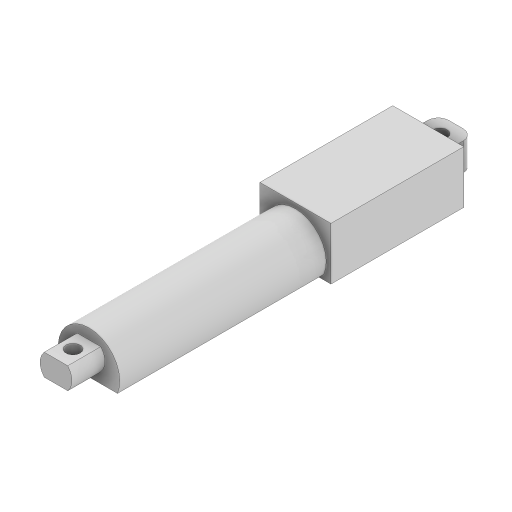
# Autodesk Inventor part: actuator
Saved by Autodesk Inventor 2023 (Build 270158000, 158)
## iProperties
Created: 2023-05-17
Part Number: actuator
Material: Generic
Document SubType Name: Modeling
Designer: Juyoung Han
Density: 1 g/cm^3
Appearance: Default
Author: Juyoung Han
Autodesk Inventor part; units mm, degrees
ref_plane "YZ Plane" through (0, 0, 0) normal (1, 0, 0) x (0, 1, 0)
ref_plane "XZ Plane" through (0, 0, 0) normal (0, 1, 0) x (-1, 0, 0)
ref_plane "XY Plane" through (0, 0, 0) normal (0, 0, 1) x (1, 0, 0)
sketch "Sketch1" plane through (0, 0, 0) normal (0, 0, 1) x (1, 0, 0)
  line L0 (0, 0) -> (20, 0)
  line L1 (20, 0) -> (20, -14.8)
  line L2 (20, -14.8) -> (0, -14.8)
  line L3 (0, -14.8) -> (0, 0)
  dimension "d0" = 20
  dimension "d1" = 14.8
  constraints: 8 end point, 2 parallel, 1 horizontal, 1 perpendicular
  measures "d0" distance of L1.end L2.end
  measures "d1" distance of L0.end L1.end
extrude "Extrusion1" add sketch "Sketch1" along normal blind 37.4
sketch "Sketch2" plane through (0, 0, 37.4) normal (0, 0, 1) x (1, 0, 0)
  line L0 (0, 0) -> (0, -14.8) projected
  line L1 (20, 0) -> (0, 0) projected
  line L2 (2, -13.4) -> (18, -13.4)
  arc A0 (18, -13.4) -> (2, -13.4) centre (10, -10.0667) ccw
  point P0 (10, -7.4)
  point P1 (10, -13.4)
  constraints: 2 end point, 2 point on circle, 1 centre point, 1 horizontal, 1 midpoint
extrude "Extrusion2" add sketch "Sketch2" along normal blind 58.1
sketch "Sketch3" plane through (0, 0, 95.5) normal (0, 0, 1) x (1, 0, 0)
  arc A0 (18, -13.4) -> (2, -13.4) centre (10, -10.0667) ccw projected
  line L0 (2, -13.4) -> (18, -13.4) projected
  line L1 (2, -13.4) -> (2, -13.4)
  line L2 (2, -13.4) -> (2, -13.4) construction
  line L3 (10, -13.4) -> (22, -13.4) construction
  line L4 (18, -13.4) -> (2, -13.4) projected
  line L5 (0, -14.8) -> (20, -14.8) projected
  line L6 (6.6913, -4.35) -> (13.3087, -4.35)
  line L7 (6.6913, -10.45) -> (13.3087, -10.45)
  arc A1 (6.6913, -4.35) -> (6.6913, -10.45) centre (10, -7.4) ccw
  arc A2 (13.3087, -10.45) -> (13.3087, -4.35) centre (10, -7.4) ccw
  point P0 (0, 0)
  dimension "d12" = 90
  constraints: 10 end point, 5 point on circle, 2 centre point, 2 horizontal, 1 midpoint, 1 perpendicular, 1 point on line
  measures "d12" angle of L2 L1
extrude "Extrusion3" add sketch "Sketch3" along normal blind 9.3 contours L6 A2 L7 A1
sketch "Sketch4" plane through (6.6913, -4.35, 95.5) normal (0, 1, 0) x (1, 0, 0)
  circle A0 centre (3.3087, -4.5) radius 2
  line L0 (-5.358, 0) -> (11.9754, 0) projected
  point P0 (-6.6913, 95.5)
  point P1 (11.3087, 0)
  point P2 (-4.6913, 0)
  dimension "d21" = 4
  dimension "d22" = 4.5
  constraints: 1 centre point
  measures "d21" diameter of A0
  measures "d22" distance from line of L0 A0.centre
extrude "Extrusion4" cut sketch "Sketch4" against normal through all
sketch "Sketch5" plane through (0, 0, 0) normal (0, 0, -1) x (-1, 0, 0)
  line L0 (-15, -3.5) -> (-5, -3.5)
  line L1 (-5, -3.5) -> (-5, -11.3)
  line L2 (-5, -11.3) -> (-15, -11.3)
  line L3 (-15, -11.3) -> (-15, -3.5)
  line L4 (-15, -3.5) -> (-5, -11.3) construction
  line L5 (-5, -3.5) -> (-15, -11.3) construction
  line L6 (-20, 0) -> (0, 0) projected
  line L7 (0, -14.8) -> (-20, -14.8) projected
  line L8 (0, 0) -> (0, -14.8) projected
  line L9 (-20, 0) -> (0, 0) projected
  line L10 (-20, -14.8) -> (-20, 0) projected
  point P0 (-10, -7.4)
  point P1 (0, -7.4)
  point P2 (-10, -7.4)
  dimension "d25" = 7.8
  dimension "d26" = 10
  dimension "d27" = 10
  constraints: 12 end point, 4 midpoint, 2 parallel, 1 horizontal, 1 perpendicular
  measures "d25" distance of L0.end L1.end
  measures "d26" distance of point (0, -7.4) point (-10, -7.4)
  measures "d27" distance of L1.end L2.end
extrude "Extrusion5" add sketch "Sketch5" along normal blind 7.8 contours L0 L1 L2 L3
sketch "Sketch6" plane through (5, -3.5, 0) normal (0, 1, 0) x (1, 0, 0)
  circle A0 centre (5, 3.3) radius 2
  line L0 (0, 7.8) -> (10, 7.8) projected
  line L1 (0, 0) -> (0, 7.8) projected
  point P0 (-5, 0)
  point P1 (5, 7.8)
  dimension "d30" = 4
  dimension "d31" = 4.5
  dimension "d32" = 5
  constraints: 1 centre point, 1 midpoint
  measures "d30" diameter of A0
  measures "d31" distance of point (5, 7.8) A0.centre
  measures "d32" distance from line of A0.centre L1
extrude "Extrusion6" cut sketch "Sketch6" against normal through all
fillet "Fillet1" radius 3 2 edges at (15, -7.4, -7.8) (5, -7.4, -7.8)
body "Solid1"
